Autodesk Fusion 360 part; units mm, degrees
(part 2 of 2)
extrude "Extrusion5" cut sketch "Skizze1 (3)" against normal blind 55 contours S0 S1 L0 S2 S3 L1 | S4 S5 S6 S7 S8 S9 S10 S11 L2 S12 S13 S14 S15 S16 S17 L3 | L4 L5 S18 S19 L6 S20 S21 S22 L7 L8 L9 L10 | S23 S24 S25 S26 L11 S27 S28 L12 | L13 L14 L15 L16 | S29 S30 S31 S32 L17 S33 S34 S35 S36 S37 S38 S39 S40 L18 | S41 S42 L19 S43 S44 S45 S46 S47 S48 S49 S50 L20 S51 S52 | S53 S54 S55 S56 S57 S58 S59 S60 S61 S62 S63 S64 S65 S66 S67 S68 S69 S70 L21 S71 S72 S73 S74 S75 S76 S77 S78 L22 S79 S80 S81 S82 S83 S84 L23 | S85 S86 S87 S88 L24 L25 L26 | S89 S90 S91 S92 S93 S94 L27 L28 L29 S95 S96 L30 | L31 L32 L33 L34 | L35 S97 S98 L36 S99 S100 S101 S102 S103 L37 L38 | S104 S105 S106 S107 L39 S108 S109 S110 S111 S112 S113 S114 S115 L40 | S116 S117 S118 L41 S119 S120 S121 L42 | S122 S123 S124 S125 L43 S126 S127 L44 | L45 L46 L47 L48 | L49 L50 L51 L52 | L53 L54 L55 L56 | L57 L58 L59 L60 L61 | S128 S129 S130 S131 L62 S132 S133 S134 S135 S136 S137 S138 S139 L63 | S140 S141 L64 S142 S143 S144 S145 S146 S147 S148 S149 L65 S150 S151 | L66 S152 S153 S154 S155 S156 S157 L67 L68 S158 S159 S160 S161 S162 S163 S164 S165 S166 S167 S168 S169 L69 | L70 L71 S170 S171 S172 S173 S174 S175 S176 S177 L72 S178 S179 S180 S181 S182 L73 | L74 L75 L76 L77 | L78 L79 L80 L81 | S183 S184 S185 S186 L82 L83 L84 S187 S188 S189 S190 L85 | L86 L87 L88 L89 | L90 L91 L92 L93 | L94 L95 L96 L97 | S191 S192 S193 S194 L98 S195 S196 S197 S198 S199 S200 S201 S202 L99 | S203 S204 L100 S205 S206 S207 S208 S209 S210 S211 S212 L101 S213 S214 | L102 L103 L104 L105 | S215 S216 S217 S218 L106 L107 L108 S219 S220 L109 | L110 L111 L112 L113 | L114 L115 L116 L117 | S221 S222 S223 S224 S225 S226 S227 S228 S229 S230 S231 L118 S232 S233 S234 S235 S236 S237 S238 S239 L119 | S240 S241 L120 S242 S243 S244 S245 S246 S247 S248 L121 S249 S250 S251 S252 S253 S254 S255 S256 | L122 S257 S258 L123 S259 S260 S261 S262 S263 L124 L125 | S264 S265 S266 S267 L126 S268 S269 S270 S271 S272 S273 S274 S275 L127 | S276 S277 S278 L128 S279 S280 S281 L129 bodies 1 in component "Tafe"
component "Tafe" placed x (1, 0, 0) y (0, 1, 0) z (0, 0, 1) at (0, 0, 0)
component "Ständer" placed x (1, 0, 0) y (0, 1, 0) z (0, 0, 1) at (0, 0, 0)
named bodies: "Grundplatte"
